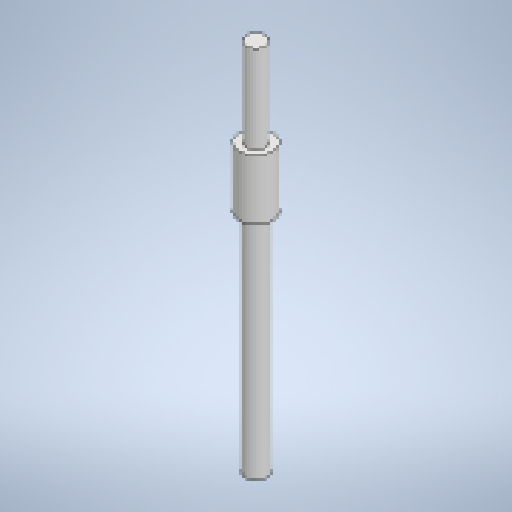
# Autodesk Inventor part: NVPH-312 augur shaft
Saved by Autodesk Inventor 2025.1 (Build 291241020, 241B)
## iProperties
Created: 2024-12-05
Part Number: NVPH-312 augur shaft
Material: Generic
Document SubType Name: Modeling
Designer: user
Density: 1 g/cm^3
Appearance: Default
Author: user
Autodesk Inventor part; units mm, degrees
ref_plane "XZ Plane" through (0, 0, 0) normal (0, 1, 0) x (-1, 0, 0)
ref_plane "XY Plane" through (0, 0, 0) normal (0, 0, 1) x (1, 0, 0)
sketch "Sketch2" plane through (0, 0, 0) normal (0, 1, 0) x (-1, 0, 0)
  line L0 (0, 0) -> (0, 513)
  line L1 (0, 513) -> (-12.5, 513)
  line L2 (-12.5, 513) -> (-12.5, 393)
  line L3 (-19, 393) -> (-19, 308)
  line L4 (-19, 308) -> (-15, 308)
  line L5 (-15, 308) -> (-15, 0)
  line L6 (-15, 0) -> (0, 0)
  line L7 (-19, 393) -> (-12.5, 393)
  dimension "d6" = 30
  dimension "d11" = 308
  dimension "d12" = 85
  dimension "d13" = 120
  dimension "d14" = 38
  dimension "d15" = 25
  constraints: 16 end point, 5 perpendicular, 1 horizontal, 1 parallel, 1 vertical
  measures "d6" diameter of L5 L0
  measures "d11" distance of L4.end L5.end
  measures "d12" distance of L3.start L3.end
  measures "d13" distance of L1.end L2.end
  measures "d14" diameter of L3 L0
  measures "d15" diameter of L2 L0
revolve "Revolution1" add sketch "Sketch2" angle 360 about axis through (0, 0, 0) along (0, 0, 1)
ref_plane "Work Plane1" through (-12.5, 0, 453) normal (1, 0, 0) x (0, 1, 0)
sketch "Sketch3" plane through (-12.5, 0, 453) normal (1, 0, 0) x (0, 1, 0)
  line L0 (12.5, -60) -> (-12.5, -60) projected
  line L1 (12.5, 60) -> (-12.5, 60) projected
  line L2 (0.1403, 48) -> (0.1403, 38) construction
  line L3 (-3.8597, 48) -> (-3.8597, 38)
  line L4 (4.1403, 38) -> (4.1403, 48)
  arc A0 (4.1403, 48) -> (-3.8597, 48) centre (0.1403, 48) ccw
  arc A1 (-3.8597, 38) -> (4.1403, 38) centre (0.1403, 38) ccw
  point P0 (0, -453)
  point P1 (0.1403, 43)
  dimension "d8" = 12
  dimension "d9" = 8
  dimension "d10" = 10
  constraints: 8 end point, 4 point on circle, 4 tangent, 2 centre point, 1 midpoint, 1 parallel, 1 perpendicular, 1 vertical
  measures "d8" distance from line of L2.start L1
  measures "d9" distance between parallel lines of L4 L3
  measures "d10" distance of L2.start L2.end
extrude "Extrusion2" cut sketch "Sketch3" along normal blind 10
body "Solid2"
